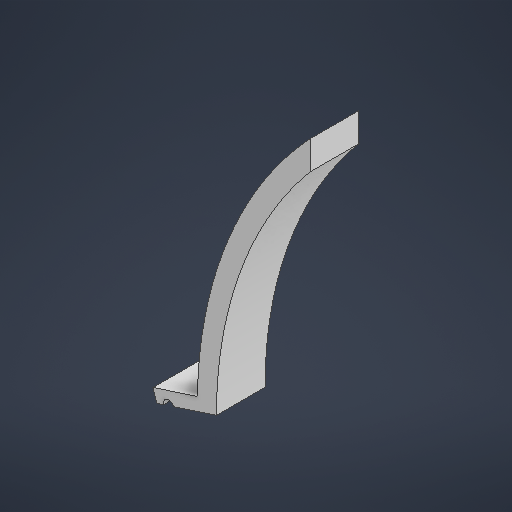
# Autodesk Inventor part: направление
Saved by Autodesk Inventor 2025 (Build 290162000, 162)
## iProperties
Created: 2025-11-04
Part Number: направление
Material: Типовые
Document SubType Name: Modeling
Designer: GameHD
Density: 1 g/cm^3
Appearance: По умолчанию
Author: GameHD
Autodesk Inventor part; units mm, degrees
ref_plane "YZ Plane" through (0, 0, 0) normal (1, 0, 0) x (0, 1, 0)
ref_plane "XZ Plane" through (0, 0, 0) normal (0, 1, 0) x (-1, 0, 0)
ref_plane "XY Plane" through (0, 0, 0) normal (0, 0, 1) x (1, 0, 0)
sketch "Эскиз1" plane through (0, 0, 0) normal (0, 0, 1) x (1, 0, 0)
  circle A0 centre (0, 0) radius 165
  circle A1 centre (0, 0) radius 172.834
  line L0 (-125, 0) -> (-126.5392, 117.7261)
  line L1 (-132.7592, 119.5177) -> (-197.8467, 76.6552)
  line L2 (-165, 0) -> (-153, 0) construction
  line L3 (-134.7038, 9.8338) -> (-172.765, -2.5204) projected
  line L4 (-165, 0) -> (-172.8154, -2.5368)
  point P0 (-172.834, 0)
  point P1 (-126.3868, 106.0725)
  point P2 (-123, 114.4334)
  point P3 (-172.8149, -2.5694)
  dimension "d0" = 330
  dimension "d1" = 345.668
  dimension "d2" = 40
  constraints: 8 end point, 4 point on circle, 2 coincident, 1 centre point, 1 collinear, 1 horizontal, 1 tangent, 3 other
  measures "d1" diameter of A1
  measures "d2" distance of L2.start L0.start
extrude "Выдавливание1" add sketch "Эскиз1" along normal blind 20 contours L3 L4 A1 L0 A0 picked at (-133.2989, 101.385)
sketch "Эскиз2" plane through (0, 0, 0) normal (0, 0, -1) x (-1, 0, 0)
  arc A0 (172.8154, -2.5368) -> (126.5392, 117.7261) centre (0, 0) ccw projected
  arc A1 (165, 0) -> (126.3868, 106.0725) centre (0, 0) ccw projected
  circle A2 centre (0, 0) radius 168.917
  line L0 (172.8154, -2.5368) -> (165, 0) projected
  circle A3 centre (184.6734, -6.3858) radius 2.1
  line L1 (178.0154, -4.2246) -> (172.8154, -2.5368)
  line L2 (160.1198, 6.946) -> (198.8648, -5.6302)
  line L3 (182.8662, -5.7992) -> (187.0032, 6.946)
  line L4 (178.0154, -4.2246) -> (198.192, -10.7737)
  line L5 (184.6734, -6.3858) -> (189.5243, -7.9603)
  line L6 (189.5243, -7.9603) -> (192.7095, 1.8528)
  point P0 (184.4408, -0.9483)
  point P1 (172.8109, 2.8266)
  point P2 (176.018, -3.5763)
  point P3 (182.676, -5.7374)
  point P4 (183.1424, -4.9484)
  point P5 (164.9119, 5.3905)
  point P6 (186.6708, -7.0341)
  point P7 (191.0988, -3.1094)
  dimension "d8" = 337.834
  dimension "d11" = 4.2
  dimension "d18" = 5.1
  constraints: 12 end point, 2 centre point, 2 perpendicular, 1 coincident, 1 collinear, 1 parallel, 1 point on line
  measures "d8" diameter of A2
  measures "d11" diameter of A3
  measures "d18" distance of L5.start L5.end
extrude "Выдавливание2" add sketch "Эскиз2" against normal up to surface (20 mm away) contours L0 A2 L2 A0 | A0 L2 L3 A3 L4 L1 | L0 A1 L2 A2 | L2 L6 L4 A3 L3 picked at (166.282, 2.7097)
